Autodesk Fusion 360 part; units mm, degrees
note: some values were not read from the file. Set by a fixed rule: which face or edge a step refers to.
(part 2 of 2)
equation "d517 = RelayBoxLidMargin"
equation "d518 = RelayBoxLidMargin"
equation "d524 = M3HoleDiameter"
equation "d525 = CarrageOffset"
equation "CarrageBoltWidth = 6.7 mm"
equation "CarrageBoltHorizontalSpace = 49 mm - CarrageBoltWidth"
equation "CarrageBoltVerticalSpace = 17 mm - CarrageBoltWidth"
equation "d533 = CarrageBoltWidth"
equation "d534 = CarrageBoltWidth"
equation "d535 = CarrageBoltWidth"
equation "d536 = CarrageBoltWidth"
equation "d537 = CarrageBoltWidth"
equation "d538 = CarrageBoltWidth"
equation "d539 = CarrageBoltWidth"
equation "d540 = CarrageBoltWidth"
equation "d541 = CarrageBoltHorizontalSpace"
equation "d542 = CarrageBoltVerticalSpace"
equation "d543 = CarrageBoltVerticalSpace"
equation "d544 = CarrageOffset"
equation "d545 = CarrageBoltHorizontalSpace"
equation "CarrageOffset = 40 mm"
equation "d547 = BoxLength / 2 - CarrageBoltVerticalSpace / 2 - CarrageBoltWidth"
equation "CarrageWasherDiameter = 20 mm"
equation "d549 = CarrageWasherDiameter"
equation "d550 = CarrageWasherDiameter"
named bodies: "ReaderBodyLeft", "LcdHousing", "ReaderBodyRight", "CardReaderFace-DontPrint", "BackLid-DontPrint", "RelayBox", "RelayBoxLid", "CarrageWasher"
